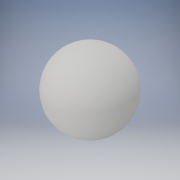
# Autodesk Inventor part: ball
Saved by Autodesk Inventor 2019 (Build 230136000, 136)
## iProperties
Created: 2019-02-18
Part Number: ball
Material: Generic
Document SubType Name: Modeling
Designer: Tesler
Density: 1 g/cm^3
Appearance: Default
Author: Tesler
Autodesk Inventor part; units mm, degrees
ref_plane "YZ Plane" through (0, 0, 0) normal (1, 0, 0) x (0, 1, 0)
ref_plane "XZ Plane" through (0, 0, 0) normal (0, 1, 0) x (-1, 0, 0)
ref_plane "XY Plane" through (0, 0, 0) normal (0, 0, 1) x (1, 0, 0)
sketch "Sketch1" plane through (0, 0, 0) normal (0, 0, 1) x (1, 0, 0)
  line L0 (0, 0) -> (0, 22.225)
  arc A0 (0, 0) -> (0, 22.225) centre (0, 11.1125) ccw
  point P0 (11.1125, 11.1125)
  dimension "d0" = 22.225
  dimension "d1" = 11.1125
  dimension "d2" = 11.1125
  constraints: 3 point on circle, 2 end point, 1 centre point, 1 vertical
  measures "d0" distance of L0.start L0.end
  measures "d1" distance from line of L0 point (11.113, 11.113)
  measures "d2" horizontal distance of point (11.113, 11.113) L0.start
revolve "Revolution1" add sketch "Sketch1" angle 360 about axis through (0, 0, 0) along (0, 1, 0)
equation "\"d2\" = d1"
body "Solid1"
